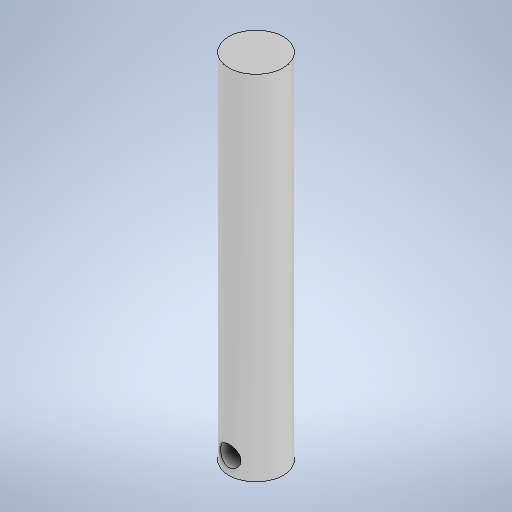
# Autodesk Inventor part: 201 part  1
Saved by Autodesk Inventor 2025.1 (Build 291241000, 241)
## iProperties
Created: 2024-08-01
Part Number: 201 part  1
Material: Aluminum 6061-AHC
Document SubType Name: Modeling
Designer: ffogue
Density: 2.7 g/cm^3
Appearance: Aluminum - Dark
Author: ffogue
Autodesk Inventor part; units mm, degrees
ref_plane "YZ Plane" through (0, 0, 0) normal (1, 0, 0) x (0, 1, 0)
ref_plane "XY Plane" through (0, 0, 0) normal (0, 0, 1) x (1, 0, 0)
sketch "Sketch1" plane through (0, 0, 0) normal (0, 0, 1) x (1, 0, 0)
  circle A0 centre (0, 0) radius 4
  dimension "d0" = 8
  constraints: 1 centre point, 1 coincident
  measures "d0" diameter of A0
extrude "Extrusion1" add sketch "Sketch1" along normal blind 52
ref_plane "Work Plane1" through (0, 4, 0) normal (0, 1, 0) x (-1, 0, 0)
sketch "Sketch2" plane through (0, 4, 0) normal (0, 1, 0) x (-1, 0, 0)
  point P0 (0, 0)
  point P1 (0, 2.5)
  dimension "d4" = 2.5
  constraints: 1 vertical alignment
  measures "d4" distance of point (0, 0) point (0, 2.5)
hole "Hole1" at (0, 4, 2.5) direction (0, -1, 0) diameter 3 end through all
body "Solid1"
